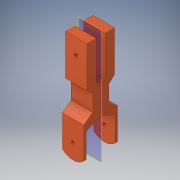
# Autodesk Inventor part: arm_m23
Saved by Autodesk Inventor 2017 (Build 210142000, 142)
## iProperties
Created: 2017-02-24
Part Number: arm_m23
Material: Phenolic Resin
Document SubType Name: Modeling
Designer: Canton
Density: 1.38 g/cm^3
Appearance: Smooth - Light Orange
Author: Canton
Autodesk Inventor part; units mm, degrees
ref_plane "YZ Plane" through (0, 0, 0) normal (1, 0, 0) x (0, 1, 0)
ref_plane "XZ Plane" through (0, 0, 0) normal (0, 1, 0) x (-1, 0, 0)
ref_plane "XY Plane" through (0, 0, 0) normal (0, 0, 1) x (1, 0, 0)
sketch "Sketch1" plane through (0, 0, 0) normal (0, 0, 1) x (1, 0, 0)
  circle A0 centre (0, 0) radius 2.75
  line L0 (0, 23.75) -> (18, 23.75)
  line L1 (18, -17.7077) -> (18, 23.75)
  line L2 (18, 23.75) -> (-18, 23.75)
  line L3 (-18, 23.75) -> (-18, -17.7077)
  arc A1 (-18, -17.7077) -> (18, -17.7077) centre (0, 0) ccw
  dimension "d3" = 5.5
  dimension "d6" = 18
  constraints: 8 end point, 2 centre point, 2 coincident, 2 point on circle, 1 parallel
  measures "d3" diameter of A0
  measures "d6" distance of L0.start L0.end
ref_plane "Work Plane1" through (-18, 23.75, 0) normal (-1, 0, 0) x (0, -1, 0)
sketch "Sketch3" plane through (-18, 23.75, 0) normal (-1, 0, 0) x (0, -1, 0)
  line L0 (-22.1236, -11) -> (-11.1236, 4)
  line L1 (-11.1236, 4) -> (0, 4)
  line L2 (-22.1236, -11) -> (-50, -11)
  line L3 (-59, -1.1) -> (-127, -1.1)
  line L4 (0, 0) -> (-10.4, -24.5)
  line L5 (-127, -17.1) -> (-127, -10.0427)
  line L6 (-59, -21.9) -> (-59, -17.1)
  line L7 (-59, -17.1) -> (-127, -17.1)
  line L8 (-10.4, -24.5) -> (-56.4, -24.5)
  line L9 (-56.4, -24.5) -> (-59, -21.9)
  line L10 (-50, -11) -> (-59, -1.1)
  line L11 (-127, -10.0427) -> (-127, -1.1)
  line L12 (-127, -1.1) -> (-127, -17.1)
  line L13 (0, 0) -> (0, 4)
  dimension "d53" = 13.5
  dimension "d56" = 16
  constraints: 28 end point, 1 parallel, 1 perpendicular, 1 vertical
  measures "d53" distance between parallel lines of L8 L2
  measures "d56" distance between parallel lines of L3 L7
extrude "Extrusion1" add sketch "Sketch3" against normal blind 36
extrude "Extrusion2" add sketch "Sketch1" along normal blind 4
sketch "Sketch5" plane through (-18, 82.75, -1.1) normal (0, 0, 1) x (1, 0, 0)
  circle A0 centre (18, -82.75) radius 2.75 projected
  circle A1 centre (18, 42.25) radius 2.75
  point P0 (18, -82.75)
  dimension "d63" = 125
  dimension "d64" = 0
  dimension "d65" = 5.5
  constraints: 1 centre point
  measures "d63" distance of A1.centre A0.centre
  measures "d64" horizontal distance of A1.centre A0.centre
  measures "d65" diameter of A1
extrude "Extrusion3" cut sketch "Sketch5" against normal blind 30 contours A1
ref_plane "Work Plane3" through (18, 34.15, -24.5) normal (0, 0, -1) x (-1, 0, 0)
mirror "Mirror1" about plane through (18, 34.15, -24.5) normal (0, 0, -1) of "Extrusion2", "Extrusion1", "Extrusion3"
body "Solid1"
